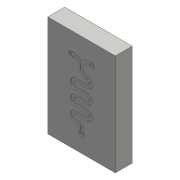
# Autodesk Inventor part: Mixer
Saved by Autodesk Inventor 2016 (Build 200138000, 138)
## iProperties
Created: 2018-10-05
Part Number: Mixer
Material: Genérico
Document SubType Name: Modeling
Designer: Joseahpacho
Density: 1 g/cm^3
Appearance: Valor por defecto
Author: Joseahpacho
Autodesk Inventor part; units mm, degrees
ref_plane "YZ Plane" through (0, 0, 0) normal (1, 0, 0) x (0, 1, 0)
ref_plane "XZ Plane" through (0, 0, 0) normal (0, 1, 0) x (-1, 0, 0)
ref_plane "XY Plane" through (0, 0, 0) normal (0, 0, 1) x (1, 0, 0)
sketch "Boceto1" plane through (0, 0, 0) normal (0, 1, 0) x (-1, 0, 0)
  line L0 (3.5954, 15.5561) -> (3.1417, 15.5533)
  line L1 (3.3005, 14.6566) -> (3.9682, 14.6566)
  line L2 (5.45, 1.7061) -> (5.45, 0.6)
  line L3 (3.5954, 15.5561) -> (4.55, 16.5107)
  line L4 (4.55, 16.5107) -> (4.55, 17.7346)
  line L5 (5.45, 17.735) -> (5.45, 16.1384)
  line L6 (5.45, 16.1384) -> (3.9682, 14.6566)
  line L7 (6.6995, 10.4566) -> (3.3005, 10.4566)
  line L8 (3.3005, 11.3566) -> (6.6995, 11.3566)
  arc A0 (6.6995, 11.3566) -> (6.6995, 12.5566) centre (6.6995, 11.9566) ccw
  arc A1 (6.6995, 10.4566) -> (6.6995, 13.4566) centre (6.6995, 11.9566) ccw
  line L9 (6.6995, 12.5566) -> (3.3005, 12.5566)
  arc A2 (3.3005, 14.6566) -> (3.3005, 13.4566) centre (3.3005, 14.0566) ccw
  arc A3 (3.1417, 15.5533) -> (3.3005, 12.5566) centre (3.3026, 14.0593) ccw
  line L10 (3.3005, 13.4566) -> (6.6995, 13.4566)
  line L11 (3.3005, 9.2566) -> (6.6995, 9.2566)
  arc A4 (3.3005, 10.4566) -> (3.3005, 9.2566) centre (3.3005, 9.8566) ccw
  arc A5 (3.3005, 11.3566) -> (3.3005, 8.3566) centre (3.3005, 9.8566) ccw
  line L12 (6.6995, 8.3566) -> (3.3005, 8.3566)
  arc A6 (6.6995, 7.1566) -> (6.6995, 8.3566) centre (6.6995, 7.7566) ccw
  arc A7 (6.6995, 6.2566) -> (6.6995, 9.2566) centre (6.6995, 7.7566) ccw
  line L13 (3.3005, 7.1566) -> (6.6995, 7.1566)
  line L14 (6.6995, 6.2566) -> (3.3005, 6.2566)
  arc A8 (3.3005, 6.2566) -> (3.3005, 5.0566) centre (3.3005, 5.6566) ccw
  arc A9 (3.3005, 7.1566) -> (3.3005, 4.1566) centre (3.3005, 5.6566) ccw
  line L15 (3.3005, 5.0566) -> (6.6995, 5.0566)
  line L16 (6.6995, 4.1566) -> (3.3005, 4.1566)
  arc A10 (6.6995, 2.9566) -> (6.6995, 4.1566) centre (6.6995, 3.5566) ccw
  arc A11 (6.6995, 2.0566) -> (6.6995, 5.0566) centre (6.6995, 3.5566) ccw
  line L17 (4.55, 2.0789) -> (5.4276, 2.9566)
  line L18 (6.6995, 2.0566) -> (5.8004, 2.0566)
  line L19 (5.8004, 2.0566) -> (5.45, 1.7061)
  line L20 (4.55, 0.6) -> (4.55, 2.0789)
  arc A12 (4.55, 0.6) -> (5.45, 0.6) centre (5, 0) ccw
  line L21 (5.4276, 2.9566) -> (6.6995, 2.9566)
  line L22 (15, -5) -> (15, 25)
  line L23 (15, 25) -> (-5, 25)
  line L24 (-5, 25) -> (-5, -5)
  line L25 (-5, -5) -> (15, -5)
  line L26 (3.7496, 18.535) -> (2.6434, 18.535)
  line L27 (4.1224, 19.435) -> (4.9998, 18.5576)
  line L28 (4.55, 17.7346) -> (3.7496, 18.535)
  line L29 (2.6434, 19.435) -> (4.1224, 19.435)
  arc A13 (2.6434, 19.435) -> (2.6434, 18.535) centre (2.0434, 18.985) ccw
  line L30 (6.2504, 18.5355) -> (7.3566, 18.5355)
  line L31 (7.3566, 19.4355) -> (5.8776, 19.4355)
  arc A14 (7.3566, 18.5355) -> (7.3566, 19.4355) centre (7.9566, 18.9855) ccw
  line L32 (5.45, 17.735) -> (6.2504, 18.5355)
  line L33 (5.8776, 19.4355) -> (4.9998, 18.5576)
  constraints: 68 end point, 30 point on circle, 15 centre point
extrude "Extrusión1" add sketch "Boceto1" along normal blind 5 contours L3 L4 L28 L26 A13 L29 L27 L33 L31 A14 L30 L32 L5 L6 L1 A2 L10 A1 L7 A4 L11 A7 L14 A8 L15 A11 L18 L19 L2 A12 L20 L17 L21 A10 L16 A9 L13 A6 L12 A5 L8 A0 L9 A3 L0 | L25 L24 L23 L22
extrude "Extrusión2" cut sketch "Boceto1" along normal blind 0.2 contours L3 L4 L28 L26 A13 L29 L27 L33 L31 A14 L30 L32 L5 L6 L1 A2 L10 A1 L7 A4 L11 A7 L14 A8 L15 A11 L18 L19 L2 A12 L20 L17 L21 A10 L16 A9 L13 A6 L12 A5 L8 A0 L9 A3 L0
sketch "Boceto3" plane through (0, 0.2, 0) normal (0, -1, 0) x (1, 0, 0)
  arc A0 (-2.6434, 18.535) -> (-2.6434, 19.435) centre (-2.0434, 18.985) ccw projected
  arc A1 (-7.3566, 19.4355) -> (-7.3566, 18.5355) centre (-7.9566, 18.9855) ccw projected
  arc A2 (-5.45, 0.6) -> (-4.55, 0.6) centre (-5, 0) ccw projected
  circle A3 centre (-2.0434, 18.985) radius 0.35
  circle A4 centre (-7.9566, 18.985) radius 0.35
  circle A5 centre (-5, 0) radius 0.35
  point P0 (0, 0)
  dimension "d5" = 0.7
  dimension "d6" = 0.7
  dimension "d7" = 0.7
  constraints: 3 centre point, 1 coincident
  measures "d5" diameter of A3
  measures "d6" diameter of A4
  measures "d7" diameter of A5
extrude "Extrusión3" cut sketch "Boceto3" against normal through all
